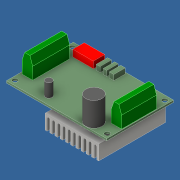
# Autodesk Inventor part: StepperDriver
Saved by Autodesk Inventor 2016 (Build 200138000, 138)
## iProperties
Created: 2016-03-01
Part Number: StepperDriver
Material: Generisch
Document SubType Name: Modeling
Designer: 4ndreas
Density: 1 g/cm^3
Appearance: Vorgabe
Mass: 30.455 g
Surface Area: 276.419 cm^2
Volume: 30.455 cm^3
Author: 4ndreas
Autodesk Inventor part; units mm, degrees
ref_plane "YZ Plane" through (0, 0, 0) normal (1, 0, 0) x (0, 1, 0)
ref_plane "XZ Plane" through (0, 0, 0) normal (0, 1, 0) x (-1, 0, 0)
ref_plane "XY Plane" through (0, 0, 0) normal (0, 0, 1) x (1, 0, 0)
sketch "Skizze1" plane through (0, 0, 0) normal (0, 0, 1) x (1, 0, 0)
  line L0 (-37.5, -25) -> (37.5, -25)
  line L1 (37.5, -25) -> (37.5, 25)
  line L2 (37.5, 25) -> (-37.5, 25)
  line L3 (-37.5, 25) -> (-37.5, -25)
  line L4 (-37.5, -25) -> (37.5, 25) construction
  line L5 (37.5, -25) -> (-37.5, 25) construction
  circle A0 centre (-34.5, 21.5) radius 1.875
  circle A1 centre (-34.5, -21.5) radius 1.875
  line L6 (-34.5, 21.5) -> (-34.5, -21.5) construction
  line L7 (-37.5, 0) -> (37.5, 0) construction
  line L8 (34.5, -21.5) -> (-34.5, -21.5) construction
  line L9 (-34.5, -21.5) -> (-34.5, 21.5) construction
  line L10 (-34.5, 21.5) -> (34.5, 21.5) construction
  line L11 (34.5, 21.5) -> (34.5, -21.5) construction
  line L12 (34.5, -21.5) -> (-34.5, 21.5) construction
  line L13 (-34.5, -21.5) -> (34.5, 21.5) construction
  circle A2 centre (34.5, 21.5) radius 1.875
  circle A3 centre (34.5, -21.5) radius 1.875
  point P0 (0, 0)
  point P1 (-34.5, 0)
  dimension "d0" = 75
  dimension "d1" = 50
  dimension "d2" = 43
  dimension "d3" = 3.75
  dimension "d4" = 69
  constraints: 28 end point, 7 midpoint, 5 parallel, 4 centre point, 3 equal radius, 2 coincident, 2 horizontal, 2 perpendicular, 1 point on line
  measures "d0" distance between parallel lines of L1 L3
  measures "d1" distance between parallel lines of L0 L2
  measures "d2" distance of L6.start L6.end
  measures "d3" diameter of A0
  measures "d4" distance of L6.start L10.end
extrude "Extrusion1" add sketch "Skizze1" along normal blind 1.5
sketch "Skizze2" plane through (0, 0, 1.5) normal (0, 0, 1) x (1, 0, 0)
  circle A0 centre (21.7096, -18.8038) radius 6.0646
  circle A1 centre (-12.0575, -18.8038) radius 2.4017
  line L0 (-28.0752, 23.7658) -> (-12.7068, 23.7658)
  line L1 (-12.7068, 23.7658) -> (-12.7068, 15.2518)
  line L2 (-12.7068, 15.2518) -> (-28.0752, 15.2518)
  line L3 (-28.0752, 15.2518) -> (-28.0752, 23.7658)
  line L4 (-36.0228, 12.8499) -> (-28.0752, 12.8499)
  line L5 (-28.0752, 12.8499) -> (-28.0752, -14.8371)
  line L6 (-28.0752, -14.8371) -> (-36.0228, -14.8371)
  line L7 (-36.0228, -14.8371) -> (-36.0228, 12.8499)
  line L8 (29.1595, 12.8499) -> (36.903, 12.8499)
  line L9 (36.903, 12.8499) -> (36.903, -13.245)
  line L10 (36.903, -13.245) -> (29.1595, -13.245)
  line L11 (29.1595, -13.245) -> (29.1595, 12.8499)
  line L12 (-10.6178, 23.7658) -> (-7.7349, 23.7658)
  line L13 (-7.7349, 23.7658) -> (-7.7349, 15.2518)
  line L14 (-7.7349, 15.2518) -> (-10.6178, 15.2518)
  line L15 (-10.6178, 15.2518) -> (-10.6178, 23.7658)
  line L16 (-5.3072, 23.7658) -> (-2.6772, 23.7658)
  line L17 (-2.6772, 23.7658) -> (-2.6772, 15.2518)
  line L18 (-2.6772, 15.2518) -> (-5.3072, 15.2518)
  line L19 (-5.3072, 15.2518) -> (-5.3072, 23.7658)
  line L20 (-0.8059, 23.7658) -> (2.5828, 23.7658)
  line L21 (2.5828, 23.7658) -> (2.5828, 15.2518)
  line L22 (2.5828, 15.2518) -> (-0.8059, 15.2518)
  line L23 (-0.8059, 15.2518) -> (-0.8059, 23.7658)
  point P0 (0, 0)
  constraints: 48 end point, 12 parallel, 6 horizontal, 6 perpendicular, 6 point on line, 2 centre point
extrude "Extrusion2" add sketch "Skizze2" along normal blind 15 separate body contours L4 L5 L6 L7 | L8 L9 L10 L11
extrude "Extrusion3" add sketch "Skizze2" along normal blind 18 separate body contours A0
extrude "Extrusion4" add sketch "Skizze2" along normal blind 10 separate body contours A1
extrude "Extrusion5" add sketch "Skizze2" along normal blind 5 separate body contours L0 L1 L2 L3
extrude "Extrusion6" add sketch "Skizze2" along normal blind 4 contours L12 L13 L14 L15 | L16 L17 L18 L19 | L20 L21 L22 L23 bodies 1
chamfer "Fase1" distance 2 distance2 6 1 edges at (-36.0228, -0.9936, 16.5) measured on face at (-33.3736, 3.6209, 16.5)
chamfer "Fase2" distance 2 distance2 6 1 edges at (-28.0752, -0.9936, 16.5) measured on face at (-32.0403, 3.6209, 16.5)
chamfer "Fase3" distance 2 distance2 6 1 edges at (29.1595, -0.1976, 16.5) measured on face at (31.7407, -4.5467, 16.5)
chamfer "Fase4" distance 2 distance2 6 1 edges at (36.903, -0.1976, 16.5) measured on face at (33.074, 4.1516, 16.5)
sketch "Skizze3" plane through (0, 0, 0) normal (0, 0, -1) x (-1, 0, 0)
  line L0 (-5.8688, -16.2438) -> (-26.3494, -16.2438)
  line L1 (-26.3494, -16.2438) -> (-26.3494, 15.757)
  line L2 (-26.3494, 15.757) -> (-5.8688, 15.757)
  line L3 (-5.8688, 15.757) -> (-5.8688, -16.2438)
  point P0 (0, 0)
  constraints: 8 end point, 2 parallel, 1 horizontal, 1 perpendicular
extrude "Extrusion7" add sketch "Skizze3" along normal blind 5 separate body
sketch "Skizze4" plane through (0, 0, -5) normal (0, 0, -1) x (-1, 0, 0)
  line L0 (-26.3494, -16.2438) -> (-26.3494, 15.757) projected
  line L1 (-26.3494, 15.757) -> (-5.8688, 15.757) projected
  line L2 (-5.8688, 15.757) -> (-5.8688, -16.2438) projected
  line L3 (-5.8688, -16.2438) -> (-26.3494, -16.2438) projected
  circle A0 centre (-34.5, -21.5) radius 1.875 projected
  circle A1 centre (-34.5, 21.5) radius 1.875 projected
  circle A2 centre (34.5, -21.5) radius 1.875 projected
  circle A3 centre (34.5, 21.5) radius 1.875 projected
  line L4 (37.5, -25) -> (-37.5, -25) projected
  line L5 (37.5, 25) -> (37.5, -25) projected
  line L6 (-37.5, 25) -> (37.5, 25) projected
  line L7 (-37.5, -25) -> (-37.5, 25) projected
  line L8 (8.5, -25) -> (-31.5, -25)
  line L9 (-31.5, -25) -> (-31.5, 25)
  line L10 (-31.5, 25) -> (8.5, 25)
  line L11 (8.5, 25) -> (8.5, -25)
  point P0 (0, 0)
  dimension "d31" = 6
  dimension "d32" = 40
  constraints: 8 end point, 2 collinear, 2 parallel, 1 horizontal, 1 perpendicular
  measures "d31" distance between parallel lines of L9 L7
  measures "d32" distance between parallel lines of L11 L9
extrude "Extrusion8" add sketch "Skizze4" along normal blind 11 contours L0 L1 L2 L3 | L4 L9 L6 L11 bodies 6
sketch "Skizze5" plane through (-8.5, 25, -5) normal (0, 1, 0) x (1, 0, 0)
  line L0 (40, 0) -> (0, 0) projected
  line L1 (40, 0) -> (40, 11) projected
  line L2 (0, 11) -> (40, 11) projected
  line L3 (0, 0) -> (0, 11) projected
  line L4 (1.4, 11) -> (3.4, 11)
  line L5 (3.4, 11) -> (3.4, 2.5)
  line L6 (2.4, 1.5) -> (2.4, 1.5)
  line L7 (1.4, 2.5) -> (1.4, 11)
  arc A0 (1.4, 2.5) -> (2.4, 1.5) centre (2.4, 2.5) ccw
  arc A1 (2.4, 1.5) -> (3.4, 2.5) centre (2.4, 2.5) ccw
  point P0 (8.5, -5)
  dimension "d35" = 1
  dimension "d36" = 1.4
  dimension "d37" = 2
  dimension "d38" = 1.5
  constraints: 8 end point, 4 point on circle, 4 tangent, 2 centre point, 2 parallel, 1 concentric, 1 horizontal, 1 perpendicular, 1 point on line
  measures "d35" radius of A0
  measures "d36" distance between parallel lines of L3 L7
  measures "d37" distance between parallel lines of L5 L7
  measures "d38" distance edge to line of A0 L0
extrude "Extrusion9" cut sketch "Skizze5" against normal through all contours L5 A1 A0 L7 L2 bodies 6
pattern_linear "Rechteckige Anordnung1" count 10 spacing 3.9 along (1, 0, 0) of "Extrusion9" bodies 6
